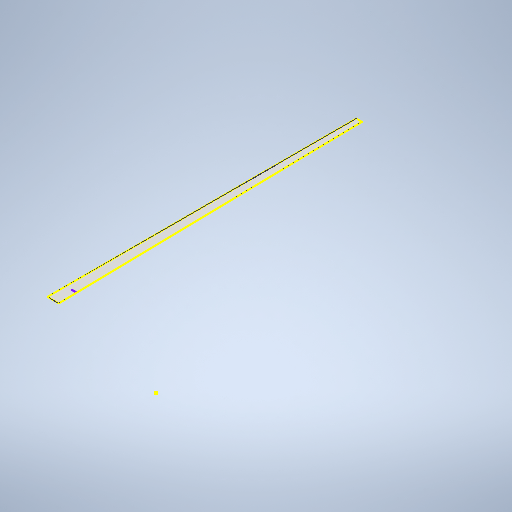
# Autodesk Inventor part: BSH 022 rib 2
Saved by Autodesk Inventor 2025 (Build 290162010, 162A)
## iProperties
Created: 2024-07-23
Part Number: BSH 022 rib 2
Material: Stainless Steel
Document SubType Name: Sheet Metal
Designer: admin
Density: 8 g/cm^3
Sheet Metal Rule: AISI304 3mm Die 32
Appearance: Default
Author: admin
Autodesk Inventor part; units mm, degrees
ref_plane "YZ Plane" through (0, 0, 0) normal (1, 0, 0) x (0, 1, 0)
ref_plane "XZ Plane" through (0, 0, 0) normal (0, 1, 0) x (-1, 0, 0)
ref_plane "XY Plane" through (0, 0, 0) normal (0, 0, 1) x (1, 0, 0)
sketch "Sketch1" plane through (0, 0, 0) normal (0, 0, 1) x (1, 0, 0)
  line L0 (1200, 2950) -> (-1200, 2950)
  line L1 (-1200, 2950) -> (-1200, 0)
  line L2 (-1200, 0) -> (1200, 0)
  line L3 (1200, 0) -> (1200, 2950)
  line L4 (1150, 2950) -> (1150, 0)
  line L5 (-1150, 0) -> (-1150, 2950) construction
  line L6 (0, 2950) -> (0, 50) construction
  line L7 (-1100, 200) -> (-950, 50)
  line L8 (-1200, 100) -> (-1100, 100)
  line L9 (-1100, 100) -> (-1100, 0)
  line L10 (-1100, 200) -> (-1150, 2950)
  arc A0 (-1100.4545, 224.9959) -> (-1082.3223, 182.3223) centre (-1100, 200) ccw
  arc A1 (-1082.3223, 182.3223) -> (-1100.4545, 224.9959) centre (-1100, 200) ccw construction
  line L11 (-1200, 255) -> (-1101, 255)
  line L12 (0, 50) -> (-950, 50)
  line L13 (0, 50) -> (0, 0)
  line L14 (1505.3449, -225.894) -> (355.3449, -225.894)
  dimension "d3" = 2400
  dimension "d4" = 2950
  dimension "d5" = 50
  dimension "d6" = 100
  dimension "d7" = 50
  dimension "d8" = 2695
  dimension "d9" = 135
  dimension "d10" = 950
  dimension "d11" = 1150
  dimension "d12" = 136.042
  dimension "d13" = 50
  dimension "d14" = 100
  dimension "d15" = 212.132
  dimension "d17" = 55
  dimension "d20" = 200
  measures "d3" distance of L3.start L1.end
  measures "d4" distance of L1.end L1.start
  measures "d5" diameter of A0
  measures "d6" distance of L8.start L8.end
  measures "d7" distance between parallel lines of L1 L5
  measures "d8" distance between parallel lines of L0 L11
  measures "d9" angle of L12 L7
  measures "d10" distance of L6.end L7.end
  measures "d11" distance of L14.start L14.end
  measures "d12" angle of L7 L10
  measures "d13" distance between parallel lines of L2 L12
  measures "d14" distance from line of L1 L10.start
  measures "d15" distance of L10.start L7.end
  measures "d17" vertical distance of L10.start L11.end
  measures "d20" distance from line of L2 A1.centre
extrude "Plate1" add sketch "Sketch1" along normal blind 3 contours L10 L11 L1 L0
sketch "Sketch2" plane through (0, 0, 3) normal (0, 0, 1) x (1, 0, 0)
  line L0 (-1101, 255) -> (-1200, 255) projected
  line L1 (-1150, 2950) -> (-1101, 255) projected
  line L2 (-1200, 2950) -> (-1150, 2950) projected
  line L3 (-1200, 255) -> (-1200, 2950) projected
  line L4 (-1101, 255) -> (-1150, 2950) projected
  line L5 (-1103.9297, 416.1313) -> (-1145.394, 415.3775)
  line L6 (-1145.394, 415.3775) -> (-1145.3392, 412.3622)
  line L7 (-1145.3392, 412.3622) -> (-1103.8748, 413.1161)
  point P0 (0, 0)
  constraints: 6 end point, 3 perpendicular, 2 point on line
equation "\"d11\" = d10 + d18"
equation "\"d14\" = d6"
equation "\"d2\" = Thickness"
equation "\"BendReliefWidth\" = Thickness"
equation "\"BendReliefDepth\" = 0.5 * Thickness"
equation "\"CornerReliefSize\" = 4 * Thickness"
equation "\"MinimumRemnant\" = 2 * Thickness"
equation "\"TransitionRadius\" = BendRadius"
equation "\"JacobiRadiusSize\" = BendRadius"
equation "\"GapSize\" = Thickness"
equation "\"d18\" = d19"
equation "\"Thickness\" = 3"
equation "\"BendRadius\" = 5"
equation "\"d19\" = 200"
body "Solid1"
